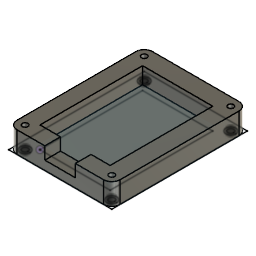
Mriduls_hackpad (Autodesk Fusion 360 design; units mm, degrees)
part number: 2025-11-27-11-23-29-888
part number: 2025-11-27-11-26-20-085
Autodesk Fusion 360 part; units mm, degrees
sketch "Sketch1" plane through (0, 0, 0) normal (0, 0, 1) x (1, 0, 0) in component "Some Fidget Keyboard"
  line L0 (0, 0) -> (42.54, 0)
  line L1 (42.54, 0) -> (42.54, 62.204)
  line L2 (42.54, 62.204) -> (0, 62.204)
  line L3 (0, 62.204) -> (0, 0)
  line L4 (-9.5, 72.704) -> (53.04, 72.704)
  line L5 (53.04, 72.704) -> (53.04, -9.5)
  line L6 (53.04, -9.5) -> (-9.5, -9.5)
  line L7 (-9.5, -9.5) -> (-9.5, 72.704)
  circle A0 centre (-4.5, 67.704) radius 1.7
  circle A1 centre (48.04, 67.704) radius 1.7
  circle A2 centre (48.04, -4.5) radius 1.7
  circle A3 centre (-4.5, -4.5) radius 1.7
  circle A4 centre (-4.5, 67.704) radius 3
  circle A5 centre (48.04, 67.704) radius 3
  circle A6 centre (48.04, -4.5) radius 3
  circle A7 centre (-4.5, -4.5) radius 3
  dimension "d4" = 42.54
  dimension "d5" = 62.204
  dimension "d6" = 62.54
  dimension "d7" = 82.204
  dimension "d8" = 9.5
  dimension "d9" = 9.5
  dimension "d10" = 3.4
  dimension "d11" = 3.4
  dimension "d12" = 3.4
  dimension "d13" = 3.4
  dimension "d14" = 5
  dimension "d15" = 5
  dimension "d16" = 5
  dimension "d17" = 5
  dimension "d18" = 5
  dimension "d20" = 5
  dimension "d21" = 5
  dimension "d22" = 5
  dimension "d23" = 6
  dimension "d24" = 6
  dimension "d25" = 6
  dimension "d26" = 6
  constraint horizontal L0
  constraint vertical L1
  constraint horizontal L2
  constraint vertical L3
  constraint coincident L0.start L3.end
  constraint horizontal L4
  constraint vertical L5
  constraint horizontal L6
  constraint vertical L7
  constraint concentric A0 A4
  constraint concentric A1 A5
  constraint concentric A2 A6
  constraint concentric A3 A7
  measures "d4" distance of L1.end L2.end
  measures "d5" distance of L0.end L1.end
  measures "d6" distance of L4.start L4.end
  measures "d7" distance of L4.start L6.end
  measures "d8" distance of L0 L6
  measures "d9" distance of L3 L7
  measures "d10" diameter of A0
  measures "d11" diameter of A1
  measures "d12" diameter of A2
  measures "d13" diameter of A3
  measures "d14" vertical distance of L4.start A0.centre
  measures "d15" horizontal distance of L4.start A0.centre
  measures "d16" vertical distance of L4.end A1.centre
  measures "d17" horizontal distance of L4.end A1.centre
  measures "d18" vertical distance of L5.end A2.centre
  measures "d20" horizontal distance of L5.end A2.centre
  measures "d21" vertical distance of L6.end A3.centre
  measures "d22" horizontal distance of L6.end A3.centre
  measures "d23" diameter of A4
  measures "d24" diameter of A5
  measures "d25" diameter of A6
  measures "d26" diameter of A7
extrude "Extrude1" add sketch "Sketch1" along normal blind 9.9 from surface at 3.1 contours A4 | A5 | A6 | A7 makes body 1 at (45.4801, 66.1397, 9.7) makes body 2 at (-7.0599, 66.1397, 9.7) makes body 3 at (51.0363, -4.6495, 9.7) makes body 4 at (-1.5037, -4.6495, 9.7) in component "Some Fidget Keyboard"
extrude "Extrude2" add sketch "Sketch1" along normal blind 13 contours L4 L5 L6 L7 bodies 1 2 3 4 in component "Some Fidget Keyboard"
extrude "Extrude3" add sketch "Sketch1" along normal blind 3 contours L0 L1 L2 L3 bodies 1 in component "Some Fidget Keyboard"
sketch "Sketch2" plane through (0, 0, 0) normal (0, 0, 1) x (1, 0, 0) in component "Some Fidget Keyboard"
sketch "Sketch3" plane through (0, 0, 13) normal (0, 0, 1) x (-1, 0, 0) in component "Some Fidget Keyboard"
  circle A0 centre (-48.04, -67.704) radius 1.7
  circle A1 centre (4.5, 4.5) radius 1.7
  line L0 (0, 0) -> (0, -62.204)
  line L1 (0, -62.204) -> (-42.54, -62.204)
  line L2 (-42.54, -62.204) -> (-42.54, 0)
  line L3 (-42.54, 0) -> (0, 0)
  line L4 (9.5, 9.5) -> (-53.04, 9.5)
  line L5 (-53.04, 9.5) -> (-53.04, -72.704)
  line L6 (-53.04, -72.704) -> (9.5, -72.704)
  line L7 (9.5, -72.704) -> (9.5, 9.5)
  circle A2 centre (4.5, -67.704) radius 1.7
  circle A3 centre (-48.04, 4.5) radius 1.7
  line L8 (-30.93, 9.5) -> (-12.43, 9.5)
  line L9 (-12.43, 9.5) -> (-12.43, 0)
  line L10 (-12.43, 0) -> (-30.93, 0)
  line L11 (-30.93, 0) -> (-30.93, 9.5)
  line L12 (-53.04, -72.704) -> (-53.04, 9.5)
  dimension "d36" = 18.5
  dimension "d37" = 22.11
  constraint horizontal L8
  constraint vertical L9
  constraint horizontal L10
  constraint vertical L11
  constraint coincident L4 L8.start
  measures "d36" distance of L8.start L8.end
  measures "d37" distance of L11 L12
extrude "Extrude4" cut sketch "Sketch3" against normal blind 7.5 contours L3 L4 L8 L9 L10 L11 bodies 1 in component "Some Fidget Keyboard"
fillet "Fillet1" radius 5 1 edges at (-9.5, -9.5, 6.5) on bodies 1 in component "Some Fidget Keyboard"
fillet "Fillet2" radius 5 1 edges at (-9.5, 72.704, 6.5) on bodies 1 in component "Some Fidget Keyboard"
fillet "Fillet3" radius 5 2 edges at (53.04, 72.704, 6.5) (53.04, -9.5, 6.5) on bodies 1 in component "Some Fidget Keyboard"
sketch "Sketch1 (2)" plane through (0, 0, 0) normal (0, 0, 1) x (1, 0, 0)
sketch "Sketch2 (2)" plane through (0, 0, 3) normal (0, 0, 1) x (-1, 0, 0)
  line L0 (0, -62.204) -> (0, 0)
  line L1 (0, 0) -> (-42.54, 0)
  line L2 (-42.54, 0) -> (-42.54, -62.204)
  line L3 (-42.54, -62.204) -> (0, -62.204)
component "Some Fidget Keyboard" placed x (1, 0, 0) y (0, 1, 0) z (0, 0, 1) at (0, 0, 0)
